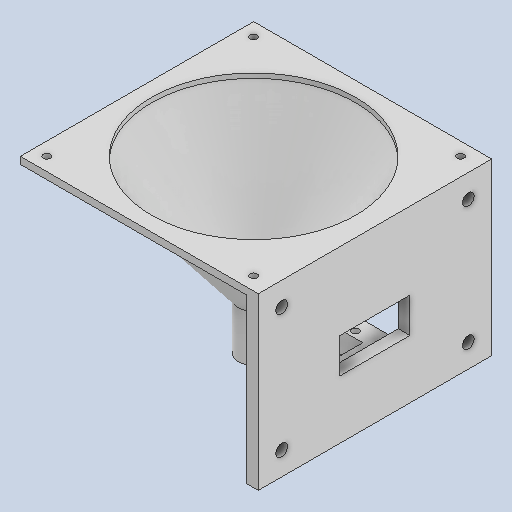
# Autodesk Inventor part: CorongBawah
Saved by Autodesk Inventor 2026.2 (Build 302298010, 298A)
## iProperties
Created: 2026-05-22
Part Number: CorongBawah
Material: Generic
Document SubType Name: Modeling
Designer: rizky
Density: 1 g/cm^3
Appearance: Default
Author: rizky
Autodesk Inventor part; units mm, degrees
ref_plane "YZ Plane" through (0, 0, 0) normal (1, 0, 0) x (0, 1, 0)
ref_plane "XY Plane" through (0, 0, 0) normal (0, 0, 1) x (1, 0, 0)
sketch "Sketch1" plane through (0, 0, 0) normal (0, 1, 0) x (-1, 0, 0)
  circle A0 centre (0, 0) radius 6
  dimension "d0" = 12
  constraints: 1 centre point, 1 coincident
  measures "d0" diameter of A0
ref_plane "Work Plane1" through (0, 50, 0) normal (0, 1, 0) x (-1, 0, 0)
sketch "Sketch2" plane through (0, 50, 0) normal (0, 1, 0) x (-1, 0, 0)
  circle A0 centre (0, 0) radius 45
  dimension "d2" = 90
  constraints: 1 centre point, 1 coincident
  measures "d2" diameter of A0
loft "Loft1" add profiles "Sketch2", "Sketch1"
shell "Shell1" thickness 2 both sides yes removed faces 1 at (-12.135255, 50, -8.816779)
sketch "Sketch3" plane through (0, 1, 0) normal (0, 1, 0) x (1, 0, 0)
  circle A0 centre (0, 0) radius 5.511773
extrude "Extrusion1" cut sketch "Sketch3" against normal through all
sketch "Sketch4" plane through (0, -1, 0) normal (0, -1, 0) x (1, 0, 0)
  circle A0 centre (0, 0) radius 5.511773
  circle A1 centre (0, 0) radius 6.488227
extrude "Extrusion2" add sketch "Sketch4" along normal blind 20
sketch "Sketch5" plane through (0, 50, 0) normal (0, 1, 0) x (1, 0, 0)
  line L0 (-50, 50) -> (50, 50)
  line L1 (50, 50) -> (50, -50)
  line L2 (50, -50) -> (-50, -50)
  line L3 (-50, -50) -> (-50, 50)
  line L4 (-50, 50) -> (50, -50) construction
  line L5 (50, 50) -> (-50, -50) construction
  line L6 (-47, -47) -> (47, -47)
  line L7 (47, -47) -> (47, 47)
  line L8 (47, 47) -> (-47, 47)
  line L9 (-47, 47) -> (-47, -47)
  circle A0 centre (0, 0) radius 43.731773
  dimension "d12" = 100
  dimension "d13" = 100
  dimension "d14" = 3
  constraints: 20 end point, 4 parallel, 2 midpoint, 2 perpendicular, 1 horizontal, 3 other
  measures "d12" distance of L1.end L2.end
  measures "d13" distance of L0.end L1.end
  measures "d14" distance between parallel lines of L2 L6
extrude "Extrusion3" add sketch "Sketch5" along normal blind 2 contours L9 L8 L7 L6
extrude "Extrusion4" add sketch "Sketch5" along normal blind 90 contours L0 L1 L2 L3
sketch "Sketch6" plane through (0, 50, 0) normal (0, -1, 0) x (1, 0, 0)
  line L0 (-50, 50) -> (50, 50)
  line L1 (-50, -50) -> (-50, 50)
  line L2 (50, -50) -> (-50, -50)
  line L3 (50, 50) -> (50, -50)
  circle A0 centre (0, 0) radius 46.268227
  line L4 (47, -47) -> (-47, -47)
  line L5 (-47, -47) -> (-47, 47)
  line L6 (-47, 47) -> (47, 47)
  line L7 (47, 47) -> (47, -47)
  point P0 (47, -13.130069)
  point P1 (13.130069, -47)
  point P2 (-13.130069, -47)
  point P3 (-47, -13.130069)
  point P4 (-47, 13.130069)
  point P5 (-13.130069, 47)
  point P6 (13.130069, 47)
  point P7 (47, 13.130069)
  dimension "d20" = 3
  constraints: 8 end point, 3 other
  measures "d20" distance between parallel lines of L3 L7
extrude "Extrusion6" add sketch "Sketch6" along normal blind 71 contours L0 L3 L2 L1
sketch "Sketch7" plane through (47, 50, -47) normal (-1, 0, 0) x (0, 0, 1)
  line L0 (94, -71) -> (0, -71) projected
  line L1 (47, -71) -> (47, -60)
  line L2 (47, -60) -> (30.3, -60)
  line L3 (30.3, -60) -> (30.3, -55)
  line L4 (30.3, -55) -> (47, -55)
  line L5 (47, -55) -> (47, -60)
  line L6 (47, -60) -> (63.7, -60)
  line L7 (63.7, -60) -> (63.7, -55)
  line L8 (63.7, -55) -> (47, -55)
  point P0 (47, -50)
  dimension "d25" = 11
  dimension "d26" = 16.7
  dimension "d27" = 5
  constraints: 16 end point, 2 parallel, 2 symmetric about line, 1 horizontal, 1 midpoint, 1 perpendicular, 1 vertical
  measures "d25" distance of L1.start L1.end
  measures "d26" distance of L3.end L4.end
  measures "d27" distance of L2.end L3.end
extrude "Extrusion8" add sketch "Sketch7" along normal blind 23.431
sketch "Sketch9" plane through (47, -10, -16.7) normal (0, -1, 0) x (1, 0, 0)
  line L0 (0, 33.4) -> (0, 0) projected
  line L1 (0, 33.4) -> (-23.431, 33.4) projected
  line L2 (-23.431, 0) -> (-23.431, 33.4) projected
  line L3 (0, 0) -> (-23.431, 0) projected
  line L4 (-23.431, 33.4) -> (-23.431, 30.7)
  line L5 (-23.431, 30.7) -> (-17.431, 30.7)
  line L6 (-23.431, 16.7) -> (-20.431, 16.7)
  circle A0 centre (-17.431, 30.7) radius 1.5
  circle A1 centre (-17.431, 2.7) radius 1.5
  point P0 (-47, 16.7)
  dimension "d32" = 2.7
  dimension "d33" = 6
  dimension "d34" = 3
  dimension "d35" = 3
  constraints: 6 end point, 2 centre point, 1 coincident, 1 horizontal, 1 midpoint, 1 perpendicular, 1 point on line, 1 symmetric about line, 1 other
  measures "d32" distance of L1.end L4.end
  measures "d33" distance of L4.end L5.end
  measures "d34" distance of L6.start L6.end
  measures "d35" diameter of A0
extrude "Extrusion9" cut sketch "Sketch9" against normal blind 5 contours A0 | A1
sketch "Sketch10" plane through (47, -10, -16.7) normal (0, -1, 0) x (1, 0, 0)
  circle A0 centre (-17.431, 2.7) radius 1.5 projected
  circle A1 centre (-17.431, 30.7) radius 1.5 projected
  line L0 (0, 33.4) -> (0, 0) projected
  line L1 (0, 33.4) -> (-23.431, 33.4) projected
  line L2 (-23.431, 0) -> (-23.431, 33.4) projected
  line L3 (0, 0) -> (-23.431, 0) projected
  line L4 (-17.431, 30.7) -> (-17.431, 27.9)
  line L5 (-17.431, 2.7) -> (-17.431, 5.5)
  line L6 (-17.431, 5.5) -> (-11.431, 5.5)
  line L7 (-11.431, 5.5) -> (-11.431, 27.9)
  line L8 (-11.431, 27.9) -> (-17.431, 27.9)
  line L9 (-17.431, 27.9) -> (-17.431, 5.5)
  line L10 (-17.431, 5.5) -> (-23.431, 5.5)
  line L11 (-23.431, 5.5) -> (-23.431, 27.9)
  line L12 (-23.431, 27.9) -> (-17.431, 27.9)
  point P0 (-47, 16.7)
  point P1 (-14.431, 5.5)
  point P2 (-23.431, 27.9)
  point P3 (-23.431, 5.5)
  dimension "d38" = 2.8
  dimension "d39" = 2.8
  dimension "d41" = 6
  dimension "d42" = 22.4
  constraints: 18 end point, 2 parallel, 2 symmetric about line, 2 vertical, 1 horizontal, 1 midpoint, 1 perpendicular
  measures "d38" distance of L4.start L4.end
  measures "d39" distance of L5.start L5.end
  measures "d41" distance between parallel lines of L9 L7
  measures "d42" distance from line of point (-14.431, 5.5) L8
extrude "Extrusion10" cut sketch "Sketch10" against normal blind 5 contours L12 L9 L10 L2 | L8 L7 L6 L9
sketch "Sketch11" plane through (47, -10, -16.7) normal (0, -1, 0) x (1, 0, 0)
  line L0 (-11.431, 5.5) -> (-23.431, 5.5) projected
  line L1 (-23.431, 0) -> (-23.431, 5.5) projected
  line L2 (0, 0) -> (-23.431, 0) projected
  line L3 (0, 33.4) -> (0, 0) projected
  line L4 (0, 33.4) -> (-23.431, 33.4) projected
  line L5 (-23.431, 27.9) -> (-23.431, 33.4) projected
  line L6 (-23.431, 27.9) -> (-11.431, 27.9) projected
  line L7 (-11.431, 27.9) -> (-11.431, 5.5) projected
  circle A0 centre (-17.431, 2.7) radius 1.5 projected
  circle A1 centre (-17.431, 30.7) radius 1.5 projected
  circle A2 centre (-17.431, 30.7) radius 2.5
  circle A3 centre (-17.431, 2.7) radius 2.5
  point P0 (-47, 16.7)
  dimension "d47" = 1
  dimension "d48" = 1
  constraints: 2 centre point
  measures "d47" radial gap between concentric circles of A1 A2
  measures "d48" radial gap between concentric circles of A0 A3
extrude "Extrusion11" add sketch "Sketch11" along normal blind 4 contours L7 L6 L5 L4 L3 L2 L1 L0
move faces "Move1" translate (0, 0, -3) faces at (31.379333, -8, -16.7)
move faces "Move2" translate (0, 0, 3) faces at (31.379333, -11, 16.7) (43.189667, -5, -4.733333)
sketch "Sketch12" plane through (50, 140, 50) normal (1, 0, 0) x (0, 0, -1)
  line L0 (100, -161) -> (100, 0) projected
  line L1 (0, 0) -> (100, 0) projected
  line L2 (0, -161) -> (0, 0) projected
  line L3 (100, -161) -> (0, -161) projected
  line L4 (50, -161) -> (50, -136)
  line L5 (50, -136) -> (35, -136)
  line L6 (35, -136) -> (35, -121)
  line L7 (35, -121) -> (50, -121)
  line L8 (50, -121) -> (50, -136)
  line L9 (50, -136) -> (65, -136)
  line L10 (65, -136) -> (65, -121)
  line L11 (65, -121) -> (50, -121)
  point P0 (50, -140)
  dimension "d55" = 25
  dimension "d56" = 15
  dimension "d57" = 15
  constraints: 16 end point, 2 parallel, 2 symmetric about line, 1 horizontal, 1 midpoint, 1 perpendicular, 1 vertical
  measures "d55" distance of L4.start L4.end
  measures "d56" distance of L6.end L7.end
  measures "d57" distance of L5.end L6.end
extrude "Extrusion12" cut sketch "Sketch12" against normal blind 3 contours L5 L6 L7 L8 | L8 L11 L10 L9
sketch "Sketch13" plane through (47, -14, -19.7) normal (0, 0, -1) x (-1, 0, 0)
  line L0 (23.431, 0) -> (0, 0) projected
  line L1 (0, 18) -> (0, 33) projected
  line L2 (0, 33) -> (0, 18) projected
  line L3 (0, 0) -> (0, 9) projected
  line L4 (0, 9) -> (0, 0) projected
  line L5 (0, 64) -> (0, -7) projected
  line L6 (0, 64) -> (0, -7) projected
  line L7 (11.7155, 0) -> (0, -7)
  point P0 (47, 14)
  point P1 (0, -7)
  constraints: 3 end point, 1 coincident, 1 midpoint
extrude "Extrusion13" add sketch "Sketch13" against normal blind 39.4
move faces "Move3" translate (0, -88, 0) faces at (49, 140, 15.666667)
sketch "Sketch14" plane through (-50, 52, 50) normal (0, 1, 0) x (1, 0, 0)
  line L0 (0, 0) -> (100, 0)
  line L1 (100, 0) -> (100, 100)
  line L2 (100, 100) -> (0, 100)
  line L3 (0, 100) -> (0, 0)
  circle A0 centre (50, 50) radius 43.731773
  line L4 (0, 0) -> (5.656854, 5.656854)
  line L5 (0, 0) -> (8, 0) construction
  circle A1 centre (5.656854, 5.656854) radius 1.5
  line L6 (0, 50) -> (3, 50)
  line L7 (50, 0) -> (50, 3)
  circle A2 centre (5.656854, 94.343146) radius 1.5
  circle A3 centre (94.343146, 5.656854) radius 1.5
  circle A4 centre (94.343146, 94.343146) radius 1.5
  dimension "d65" = 8
  dimension "d66" = 45
  dimension "d67" = 3
  dimension "d68" = 3
  dimension "d69" = 3
  constraints: 8 end point, 4 centre point, 3 symmetric about line, 2 horizontal, 2 midpoint, 1 coincident, 1 equal length, 1 vertical, 3 other
  measures "d65" distance of L0.start L4.end
  measures "d66" angle of L5 L4
  measures "d67" diameter of A1
  measures "d68" distance of L6.start L6.end
  measures "d69" distance of L7.start L7.end
extrude "Extrusion14" cut sketch "Sketch14" against normal blind 3 contours A1 | A2 | A3 | A4
sketch "Sketch16" plane through (-50, 52, 50) normal (0, 1, 0) x (1, 0, 0)
  line L0 (2.5, 97.5) -> (97.5, 97.5)
  line L1 (97.5, 97.5) -> (97.5, 2.5)
  line L2 (97.5, 2.5) -> (2.5, 2.5)
  line L3 (2.5, 2.5) -> (2.5, 97.5)
  line L4 (2.5, 97.5) -> (97.5, 2.5) construction
  line L5 (97.5, 97.5) -> (2.5, 2.5) construction
  point P0 (50, 50)
  dimension "d74" = 95
  dimension "d75" = 95
  constraints: 12 end point, 2 midpoint, 2 parallel, 1 horizontal, 1 perpendicular
  measures "d74" distance of L1.end L2.end
  measures "d75" distance of L0.end L1.end
move faces "Move4" translate (0, -1, 0) faces at (-33.064884, 50, -39.047763)
sketch "Sketch17" plane through (-50, -21, 50) normal (0, 0, 1) x (1, 0, 0)
  line L0 (100, 0) -> (100, 73) projected
  line L1 (0, 73) -> (100, 73) projected
  line L2 (0, 73) -> (0, 0) projected
  line L3 (100, 0) -> (0, 0) projected
  line L4 (97, 70) -> (97, 3)
  line L5 (97, 3) -> (3, 3)
  line L6 (3, 3) -> (3, 70)
  line L7 (3, 70) -> (97, 70)
  line L8 (97, 0) -> (97, 3)
  line L9 (0, 70) -> (3, 70)
  point P0 (50, 21)
  dimension "d79" = 3
  constraints: 12 end point, 2 point on line, 1 collinear, 1 perpendicular, 3 other
  measures "d79" distance between parallel lines of L1 L7
extrude "Extrusion15" cut sketch "Sketch17" against normal blind 3 contours L3 L2 L9 L6 L5 L8 | L5 L6 L7 L4
chamfer "Chamfer1" distance 9 angle 45 1 edges at (47, -5, 0)
sketch "Sketch18" plane through (50, -21, -50) normal (0, 0, -1) x (-1, 0, 0)
  line L0 (100, 0) -> (100, 73) projected
  line L1 (0, 73) -> (100, 73) projected
  line L2 (0, 0) -> (0, 73) projected
  line L3 (100, 0) -> (0, 0) projected
  line L4 (97, 70) -> (97, 3)
  line L5 (97, 3) -> (3, 3)
  line L6 (3, 3) -> (3, 70)
  line L7 (3, 70) -> (97, 70)
  line L8 (3, 0) -> (3, 3)
  line L9 (100, 70) -> (97, 70)
  point P0 (50, 21)
  dimension "d85" = 3
  constraints: 12 end point, 2 point on line, 1 horizontal, 1 perpendicular, 3 other
  measures "d85" distance between parallel lines of L1 L7
extrude "Extrusion16" cut sketch "Sketch18" against normal blind 3 contours L3 L8 L5 L4 L9 L0 | L4 L5 L6 L7
sketch "Sketch19" plane through (-50, 52, -50) normal (-1, 0, 0) x (0, 0, 1)
  line L0 (0, -3) -> (3, -3) projected
  line L1 (3, -3) -> (3, -73) projected
  line L2 (97, -73) -> (3, -73) projected
  line L3 (97, -73) -> (97, -3) projected
  line L4 (97, -3) -> (100, -3) projected
  line L5 (100, 0) -> (100, -3) projected
  line L6 (0, 0) -> (100, 0) projected
  line L7 (0, -3) -> (0, 0) projected
  line L8 (3, -3) -> (97, -3)
  point P0 (50, -52)
  constraints: 2 end point, 1 parallel
extrude "Extrusion17" cut sketch "Sketch19" against normal blind 3 contours L8 L3 L2 L1
move faces "Move5" translate (2, 0, 0) faces at (50, 41, -5)
sketch "Sketch21" plane through (52, -21, -50) normal (1, 0, 0) x (0, 0, -1)
  line L0 (-35, 25) -> (-65, 25) projected
  line L1 (-65, 25) -> (-65, 40) projected
  line L2 (-65, 40) -> (-35, 40) projected
  line L3 (-35, 40) -> (-35, 25) projected
  line L4 (0, 0) -> (0, 73) projected
  line L5 (-100, 73) -> (0, 73) projected
  line L6 (-100, 0) -> (-100, 73) projected
  line L7 (0, 0) -> (-100, 0) projected
  line L8 (-100, 73) -> (-90, 73)
  line L9 (-90, 73) -> (-90, 63)
  line L10 (-50, 73) -> (-50, 68)
  circle A0 centre (-90, 63) radius 2.5
  circle A1 centre (-10, 63) radius 2.5
  line L11 (-100, 36.5) -> (-95, 36.5)
  circle A2 centre (-90, 10) radius 2.5
  circle A3 centre (-10, 10) radius 2.5
  point P0 (-50, 21)
  dimension "d99" = 10
  dimension "d100" = 10
  dimension "d101" = 5
  dimension "d102" = 5
  dimension "d103" = 5
  constraints: 8 end point, 4 centre point, 3 symmetric about line, 2 midpoint, 1 coincident, 1 horizontal, 1 perpendicular, 1 point on line, 1 vertical, 3 other
  measures "d99" distance of L5.start L8.end
  measures "d100" distance of L8.end L9.end
  measures "d101" distance of L10.start L10.end
  measures "d102" diameter of A0
  measures "d103" distance of L11.start L11.end
extrude "Extrusion19" cut sketch "Sketch21" against normal blind 5 contours A0 | A1 | A2 | A3
body "Solid1"
